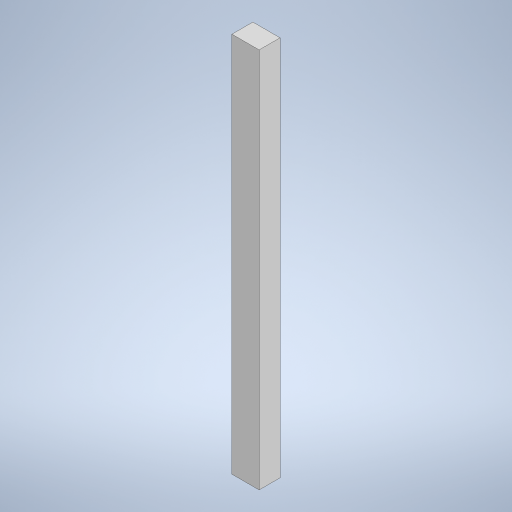
# Autodesk Inventor part: DrumstickBoundingBox
Saved by Autodesk Inventor 2023 (Build 270158000, 158)
## iProperties
Created: 2023-03-19
Part Number: DrumstickBoundingBox
Material: Generic
Document SubType Name: Modeling
Designer: valer
Density: 1 g/cm^3
Appearance: Default
Author: valer
Autodesk Inventor part; units mm, degrees
ref_plane "YZ Plane" through (0, 0, 0) normal (1, 0, 0) x (0, 1, 0)
ref_plane "XZ Plane" through (0, 0, 0) normal (0, 1, 0) x (-1, 0, 0)
ref_plane "XY Plane" through (0, 0, 0) normal (0, 0, 1) x (1, 0, 0)
sketch "BoundingBox" plane through (0, 0, 0) normal (0, 0, 1) x (1, 0, 0)
  line L0 (2.0737, -90.0906) -> (30.6487, -90.0906)
  line L1 (30.6487, -90.0906) -> (30.6487, 309.9594)
  line L2 (30.6487, 309.9594) -> (2.0737, 309.9594)
  line L3 (2.0737, 309.9594) -> (2.0737, -90.0906)
  line L4 (30.6487, -4.6434) -> (2.0737, -4.6434)
  line L5 (14.7737, 309.9594) -> (17.9487, 309.9594)
  line L6 (13.1852, -90.0906) -> (19.5373, -90.0906)
  point P0 (0, 0)
  point P1 (16.2898, -4.6434)
  point P2 (16.4327, -4.6434)
  point P3 (14.0764, -90.0906)
  point P4 (0, 0)
  constraints: 14 end point, 2 collinear, 2 parallel, 2 point on line, 1 horizontal, 1 perpendicular
extrude "BoundingBoxFeature" add sketch "BoundingBox" along normal blind 22
body "Solid1"
